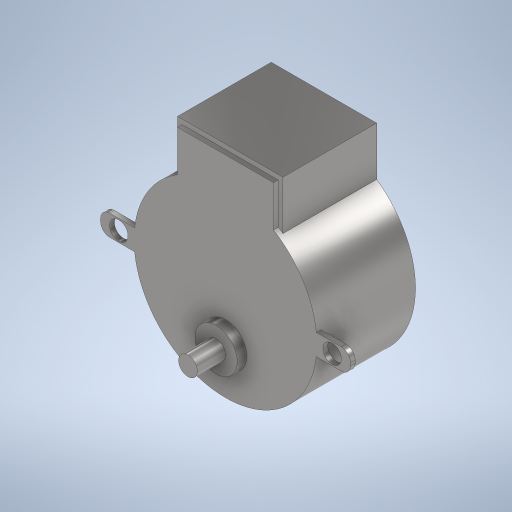
# Autodesk Inventor part: stepper_motor
Saved by Autodesk Inventor 2024.3 (Build 283343000, 343)
## iProperties
Created: 2024-06-01
Part Number: stepper_motor
Material: Acero, suave
Document SubType Name: Modeling
Designer: riera
Density: 7.85 g/cm^3
Appearance: Semipulido
Author: riera
Autodesk Inventor part; units mm, degrees
ref_plane "YZ Plane" through (0, 0, 0) normal (1, 0, 0) x (0, 1, 0)
ref_plane "XZ Plane" through (0, 0, 0) normal (0, 1, 0) x (-1, 0, 0)
ref_plane "XY Plane" through (0, 0, 0) normal (0, 0, 1) x (1, 0, 0)
sketch "Boceto1" plane through (0, 0, 0) normal (0, 0, 1) x (1, 0, 0)
  circle A0 centre (-11.375, 0) radius 0.975
  arc A1 (13.3142, 0.145) -> (12.3392, 1.12) centre (12.3392, 0.145) ccw
  line L0 (12.3392, 1.12) -> (9.6855, 1.12)
  line L1 (18.4935, 0) -> (-19.3273, 0)
  arc A2 (12.3392, -1.12) -> (13.3142, -0.145) centre (12.3392, -0.145) ccw
  line L2 (12.3392, -1.12) -> (9.6855, -1.12)
  line L3 (0, 0) -> (0, 1.0605)
  arc A3 (-12.3392, 1.12) -> (-13.3142, 0.145) centre (-12.3392, 0.145) ccw
  line L4 (-12.3392, 1.12) -> (-9.6855, 1.12)
  line L5 (-12.3392, -1.12) -> (-9.6855, -1.12)
  arc A4 (-13.3142, -0.145) -> (-12.3392, -1.12) centre (-12.3392, -0.145) ccw
  line L6 (-5.1219, 12.666) -> (5.1219, 12.666)
  arc A5 (-5.1219, 8.2963) -> (-9.6855, 1.12) centre (0, 0) ccw
  arc A6 (-9.6855, -1.12) -> (9.6855, -1.12) centre (0, 0) ccw
  arc A7 (9.6855, 1.12) -> (5.1219, 8.2963) centre (0, 0) ccw
  line L7 (-5.1219, 12.666) -> (-5.1219, 8.2963)
  line L8 (5.1219, 12.666) -> (5.1219, 8.2963)
  line L9 (-13.3142, 0.145) -> (-13.3142, -0.145)
  line L10 (13.3142, 0.145) -> (13.3142, -0.145)
  circle A8 centre (11.375, 0) radius 0.975
  point P0 (13.3033, 0)
  point P1 (13.3142, 0)
  point P2 (5.1219, 10.4811)
  dimension "d2" = 1.95
  dimension "d4" = 11.375
  dimension "d7" = 1.95
  dimension "d12" = 2.6537
  dimension "d20" = 9.75
  dimension "d21" = 2.24
  dimension "d22" = 12.666
  dimension "d24" = 10.2439
  dimension "d25" = 10.2439
  dimension "d26" = 4.3697
  dimension "d29" = 1.95
  dimension "d30" = 11.375
  constraints: 22 end point, 14 point on circle, 11 symmetric about line, 9 centre point, 4 vertical, 2 horizontal, 2 horizontal alignment, 2 point on line, 2 tangent, 1 coincident, 1 midpoint, 1 parallel, 3 other
  measures "d2" diameter of A0
  measures "d4" distance of point (0, 0) A0.centre
  measures "d7" diameter of A1
  measures "d12" distance of L2.end L2.start
  measures "d20" radius of A5
  measures "d21" diameter of L5.end L1
  measures "d22" distance from line of L6 point (0, 0)
  measures "d24" distance from line of point (5.122, 10.481) L7
  measures "d25" distance of L6.start L6.end
  measures "d26" distance of L6.end L8.end
  measures "d29" diameter of A8
  measures "d30" distance of point (0, 0) A8.centre
extrude "Extrusión3" add sketch "Boceto1" along normal blind 0.5 contours L1 A8 L10 A2 L2 A6 L5 A4 L9 A0 | A0 L1 L9 A3 L4 A5 L7 L6 L8 A7 L0 A1 L10 A8
sketch "Boceto2" plane through (0, 0, 0) normal (0, 0, -1) x (-1, 0, 0)
  line L0 (-5.1219, 12.666) -> (5.1219, 12.666) projected
  line L1 (-5.1219, 8.2963) -> (-5.1219, 12.666) projected
  arc A0 (-5.1219, 8.2963) -> (-9.6855, 1.12) centre (0, 0) ccw projected
  line L2 (-12.3392, 1.12) -> (-9.6855, 1.12) projected
  arc A1 (-12.3392, 1.12) -> (-13.3142, 0.145) centre (-12.3392, 0.145) ccw projected
  line L3 (-13.3142, -0.145) -> (-13.3142, 0.145) projected
  arc A2 (-13.3142, -0.145) -> (-12.3392, -1.12) centre (-12.3392, -0.145) ccw projected
  line L4 (-9.6855, -1.12) -> (-12.3392, -1.12) projected
  arc A3 (-9.6855, -1.12) -> (9.6855, -1.12) centre (0, 0) ccw projected
  line L5 (12.3392, -1.12) -> (9.6855, -1.12) projected
  arc A4 (12.3392, -1.12) -> (13.3142, -0.145) centre (12.3392, -0.145) ccw projected
  line L6 (13.3142, 0.145) -> (13.3142, -0.145) projected
  arc A5 (13.3142, 0.145) -> (12.3392, 1.12) centre (12.3392, 0.145) ccw projected
  line L7 (9.6855, 1.12) -> (12.3392, 1.12) projected
  arc A6 (9.6855, 1.12) -> (5.1219, 8.2963) centre (0, 0) ccw projected
  line L8 (5.1219, 12.666) -> (5.1219, 8.2963) projected
  arc A7 (-5.1219, 8.2963) -> (5.1219, 8.2963) centre (0, 0) ccw
  line L9 (-5.1219, 8.2963) -> (-5.1219, 12.666) projected
  line L10 (-5.1219, 8.2963) -> (-5.1219, 12.666)
  line L11 (-5.1219, 12.666) -> (5.1219, 12.666)
  line L12 (5.1219, 8.2963) -> (5.1219, 12.666)
  point P0 (9.6855, -1.12)
  point P1 (-9.6855, 1.12)
  constraints: 6 end point, 3 collinear, 2 point on circle, 1 centre point, 1 coincident, 1 concentric
extrude "Extrusión4" add sketch "Boceto2" along normal blind 10 contours L0 L8 A6 A7 A3 A0 L1
sketch "Boceto3" plane through (0, 0, 0) normal (0, 0, -1) x (-1, 0, 0)
  arc A0 (-5.1219, 8.2963) -> (5.1219, 8.2963) centre (0, 0) ccw projected
  line L0 (5.6225, 13.166) -> (-5.6225, 13.166)
  arc A1 (5.6225, 7.9656) -> (-5.6225, 7.9656) centre (0, 0) ccw
  line L1 (5.1219, 12.666) -> (-5.1219, 12.666) projected
  line L2 (5.6225, 13.166) -> (5.6225, 7.9656)
  line L3 (-5.6225, 13.166) -> (-5.6225, 7.9656)
  point P0 (0, 13.166)
  point P1 (0, 12.666)
  point P2 (-5.6225, 7.9656)
  point P3 (-5.1219, 8.2963)
  point P4 (5.1219, 8.2963)
  point P5 (5.6225, 7.9656)
  dimension "d38" = 11.245
  dimension "d39" = 13.166
  constraints: 6 end point, 2 midpoint, 2 point on circle, 1 centre point, 1 coincident, 1 concentric, 1 horizontal, 1 parallel, 1 vertical, 1 vertical alignment
  measures "d38" distance of L0.start L0.end
  measures "d39" distance from line of point (0, 0) L0
extrude "Extrusión6" add sketch "Boceto3" along normal blind 10 contours A0 L3 L0 L2 A1
sketch "Boceto4" plane through (0, 0, 0.5) normal (0, 0, 1) x (1, 0, 0)
  circle A0 centre (0, -4.8124) radius 2.25
  point P0 (0, 0)
  dimension "d42" = 4.5
  constraints: 1 centre point
  measures "d42" diameter of A0
extrude "Extrusión7" add sketch "Boceto4" along normal blind 1
sketch "Boceto5" plane through (0, -4.8124, 1.5) normal (0, 0, 1) x (1, 0, 0)
  circle A0 centre (0, 0) radius 1
  point P0 (0, 4.8124)
  dimension "d45" = 2
  constraints: 1 centre point
  measures "d45" diameter of A0
extrude "Extrusión8" add sketch "Boceto5" along normal blind 3
